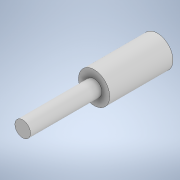
# Autodesk Inventor part: fuckup fixer
Saved by Autodesk Inventor 2022 (Build 260153000, 153)
## iProperties
Created: 2022-05-11
Part Number: fuckup fixer
Material: Generic
Document SubType Name: Modeling
Designer: erasm
Density: 1 g/cm^3
Appearance: Default
Author: erasm
Autodesk Inventor part; units mm, degrees
ref_plane "YZ Plane" through (0, 0, 0) normal (1, 0, 0) x (0, 1, 0)
ref_plane "XZ Plane" through (0, 0, 0) normal (0, 1, 0) x (-1, 0, 0)
ref_plane "XY Plane" through (0, 0, 0) normal (0, 0, 1) x (1, 0, 0)
sketch "Sketch1" plane through (0, 0, 0) normal (0, 0, 1) x (1, 0, 0)
  circle A0 centre (19, -27.5) radius 3 projected
  circle A1 centre (19, -27.5) radius 6
  point P0 (0, 0)
  dimension "d0" = 12
  constraints: 1 centre point, 1 coincident
  measures "d0" diameter of A1
extrude "Extrusion1" add sketch "Sketch1" along normal blind 24.2875
sketch "Sketch2" plane through (19, -27.5, 24.2875) normal (0, 0, 1) x (1, 0, 0)
  circle A0 centre (0, 0) radius 3
  point P0 (-19, 27.5)
  dimension "d3" = 6
  constraints: 1 centre point
  measures "d3" diameter of A0
extrude "Extrusion2" add sketch "Sketch2" along normal blind 27.4625
sketch "Sketch3" plane through (19, -27.5, 24.2875) normal (0, 0, -1) x (-1, 0, 0)
  circle A0 centre (0, 0) radius 3
  point P0 (19, 27.5)
  constraints: 1 centre point
extrude "Extrusion3" add sketch "Sketch3" along normal blind 10
body "Solid1"
